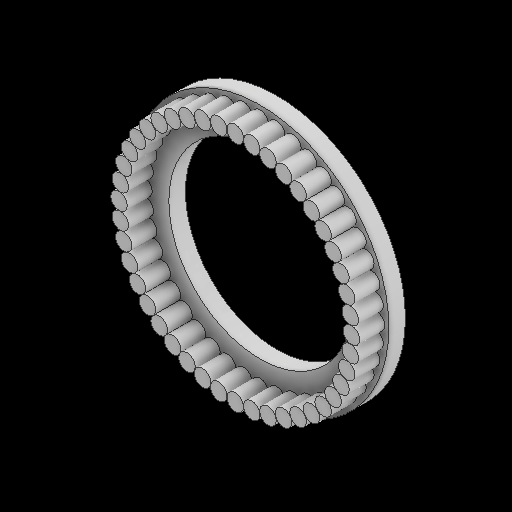
# Autodesk Inventor part: housing
Saved by Autodesk Inventor 2026 (Build 300175050, 175E)
## iProperties
Created: 2026-06-07
Part Number: housing
Material: 일반
Document SubType Name: Modeling
Designer: iamma
Density: 1 g/cm^3
Appearance: 기본값
Author: iamma
Autodesk Inventor part; units mm, degrees
ref_plane "YZ Plane" through (0, 0, 0) normal (1, 0, 0) x (0, 1, 0)
ref_plane "XZ Plane" through (0, 0, 0) normal (0, 1, 0) x (-1, 0, 0)
ref_plane "XY Plane" through (0, 0, 0) normal (0, 0, 1) x (1, 0, 0)
sketch "스케치1" plane through (0, 0, 0) normal (0, 0, 1) x (1, 0, 0)
  circle A0 centre (0, 0) radius 77.5
  dimension "d0" = 155
  constraints: 1 centre point, 1 coincident
  measures "d0" diameter of A0
extrude "돌출1" add sketch "스케치1" along normal blind 10
sketch "스케치2" plane through (0, 0, 10) normal (0, 0, 1) x (1, 0, 0)
  circle A0 centre (0, 0) radius 70 construction
  line L0 (0, 0) -> (0, 70) construction
  circle A1 centre (0, 70) radius 4.995
  dimension "d3" = 140
  dimension "d4" = 9.99
  constraints: 2 coincident, 2 end point, 1 centre point, 1 vertical, 1 vertical alignment, 2 other
  measures "d4" diameter of A1
extrude "돌출2" add sketch "스케치2" along normal blind 15
pattern_circular "원형 패턴1" count 44 over 360 about axis through (0, 0, 0) along (0, 0, 1) of "돌출2"
sketch "스케치3" plane through (0, 0, 10) normal (0, 0, 1) x (1, 0, 0)
  circle A0 centre (0, 0) radius 55
  dimension "d10" = 110
  constraints: 1 centre point, 1 coincident
  measures "d10" diameter of A0
extrude "돌출3" cut sketch "스케치3" against normal up to surface (10 mm away)
